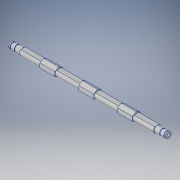
# Autodesk Inventor part: Storage Axle
Saved by Autodesk Inventor 2019.4 (Build 234330000, 330)
## iProperties
Created: 2020-01-27
Part Number: Storage Axle
Material: Aluminum 6061
Document SubType Name: Modeling
Designer: admin
Density: 2.7 g/cm^3
Appearance: Aluminum - Flat
Author: admin
Autodesk Inventor part; units mm, degrees
ref_plane "YZ Plane" through (0, 0, 0) normal (1, 0, 0) x (0, 1, 0)
ref_plane "XZ Plane" through (0, 0, 0) normal (0, 1, 0) x (-1, 0, 0)
ref_plane "XY Plane" through (0, 0, 0) normal (0, 0, 1) x (1, 0, 0)
sketch "Sketch1" plane through (0, 0, 0) normal (0, 0, 1) x (1, 0, 0)
  line L0 (0, 0) -> (0, 5)
  line L1 (19.1, 5) -> (19.1, 6)
  line L2 (19.1, 6) -> (245.3, 6)
  line L3 (245.3, 6) -> (245.3, 5)
  line L4 (264.4, 5) -> (264.4, 0)
  line L5 (264.4, 0) -> (0, 0)
  line L6 (19.1, 5) -> (10.2, 5)
  line L7 (10.2, 5) -> (10.2, 4.65)
  line L8 (10.2, 4.65) -> (9.1, 4.65)
  line L9 (9.1, 4.65) -> (9.1, 5)
  line L10 (9.1, 5) -> (3.1, 5)
  line L11 (3.1, 5) -> (3.1, 4.65)
  line L12 (3.1, 4.65) -> (2, 4.65)
  line L13 (2, 4.65) -> (2, 5)
  line L14 (2, 5) -> (0, 5)
  line L15 (245.3, 5) -> (254.2, 5)
  line L16 (254.2, 5) -> (254.2, 4.65)
  line L17 (254.2, 4.65) -> (255.3, 4.65)
  line L18 (255.3, 4.65) -> (255.3, 5)
  line L19 (255.3, 5) -> (261.3, 5)
  line L20 (261.3, 5) -> (261.3, 4.65)
  line L21 (261.3, 4.65) -> (262.4, 4.65)
  line L22 (262.4, 4.65) -> (262.4, 5)
  line L23 (262.4, 5) -> (264.4, 5)
  dimension "d1" = 6
  dimension "d2" = 226.2
  dimension "d16" = 1.1
  dimension "d17" = 1.1
  dimension "d18" = 0.35
  dimension "d19" = 10
  dimension "d20" = 16
  dimension "d21" = 2
  dimension "d22" = 5
  dimension "d23" = 1.1
  dimension "d24" = 1.1
  dimension "d25" = 0.35
  dimension "d26" = 5
  dimension "d27" = 10
  dimension "d28" = 16
  dimension "d29" = 2
  constraints: 48 end point, 15 perpendicular, 10 point on line, 2 horizontal, 1 vertical
  measures "d1" distance between parallel lines of L5 L2
  measures "d2" distance of L1.end L2.end
  measures "d16" distance of L11.end L12.end
  measures "d17" distance of L7.end L8.end
  measures "d18" distance of L6.end L7.end
  measures "d19" distance between parallel lines of L1 L9
  measures "d20" distance between parallel lines of L1 L11
  measures "d21" distance of L13.end L0.end
  measures "d22" distance between parallel lines of L5 L6
  measures "d23" distance of L16.end L17.end
  measures "d24" distance of L20.end L21.end
  measures "d25" distance of L17.end L18.end
  measures "d26" distance between parallel lines of L5 L15
  measures "d27" distance between parallel lines of L3 L18
  measures "d28" distance between parallel lines of L3 L20
  measures "d29" distance of L22.end L4.start
revolve "Revolution1" add sketch "Sketch1" angle 360 about axis through (264.4, 0, 0) along (-1, 0, 0)
sketch "Sketch2" plane through (245.3, 0, 0) normal (1, 0, 0) x (0, 0, -1)
  line L0 (-3.9686, 4.5) -> (3.9686, 4.5)
  circle A0 centre (0, 0) radius 6 projected
  point P0 (0, 0)
  dimension "d6" = 4.5
  constraints: 2 end point, 2 point on circle, 1 horizontal
  measures "d6" distance from line of A0.centre L0
extrude "Extrusion1" cut sketch "Sketch2" against normal up to surface (226.2 mm away) contours A0 L0 picked at (0, 5)
sketch "Sketch3" plane through (264.4, 0, 0) normal (1, 0, 0) x (0, 0, -1)
  circle A0 centre (0, 0) radius 5 projected
  point P0 (0, 0)
  constraints: 1 coincident
hole "Hole1" at (264.4, 0, 0) direction (-1, 0, 0) diameter 5 end through all
ref_plane "Work Plane1" through (132.2, 0, 0) normal (-1, 0, 0) x (0, 0, 1)
sketch "Sketch4" plane through (132.2, 0, 0) normal (-1, 0, 0) x (0, 0, 1)
  line L0 (0, 7.3323) -> (6.35, 3.6662)
  line L1 (6.35, 3.6662) -> (6.35, -3.6662)
  line L2 (6.35, -3.6662) -> (0, -7.3323)
  line L3 (0, -7.3323) -> (-6.35, -3.6662)
  line L4 (-6.35, -3.6662) -> (-6.35, 3.6662)
  line L5 (-6.35, 3.6662) -> (0, 7.3323)
  point P0 (0, 0)
  point P1 (0, 0)
  dimension "d30" = 12.7
  constraints: 12 end point, 1 coincident, 1 vertical, 13 other
  measures "d30" distance between parallel lines of L4 L1
extrude "Extrusion2" add sketch "Sketch4" along normal mid plane 25.4
ref_plane "Work Plane2" through (184.9, 0, 0) normal (1, 0, 0) x (0, 0, -1)
sketch "Sketch5" plane through (184.9, 0, 0) normal (1, 0, 0) x (0, 0, -1)
  line L0 (0, 7.3323) -> (-6.35, 3.6662) projected
  line L1 (-6.35, 3.6662) -> (-6.35, -3.6662) projected
  line L2 (-6.35, -3.6662) -> (0, -7.3323) projected
  line L3 (0, -7.3323) -> (6.35, -3.6662) projected
  line L4 (6.35, -3.6662) -> (6.35, 3.6662) projected
  line L5 (6.35, 3.6662) -> (0, 7.3323) projected
  line L6 (3.9686, 4.5) -> (-3.9686, 4.5) projected
  arc A0 (-3.9686, 4.5) -> (3.9686, 4.5) centre (0, 0) ccw projected
  point P0 (0, 0)
extrude "Extrusion3" add sketch "Sketch5" along normal blind 25.4
mirror "Mirror1" about plane through (132.2, 0, 0) normal (-1, 0, 0) of "Extrusion3"
body "Solid1"
